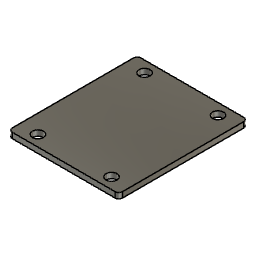
Pos34 (Autodesk Fusion 360 design; units mm, degrees)
Autodesk Fusion 360 part; units mm, degrees
sketch "Sketch1" plane through (0, 0, 0) normal (0, 0, 1) x (1, 0, 0)
  line L0 (28, -35) -> (-28, -35)
  line L1 (-30, -33) -> (-30, 33)
  line L2 (-28, 35) -> (28, 35)
  line L3 (30, 33) -> (30, -33)
  line L4 (30, -35) -> (-30, 35) construction
  line L5 (-30, -35) -> (30, 35) construction
  arc A0 (-28, 35) -> (-30, 33) centre (-28, 33) ccw
  arc A1 (30, 33) -> (28, 35) centre (28, 33) ccw
  arc A2 (28, -35) -> (30, -33) centre (28, -33) ccw
  arc A3 (-30, -33) -> (-28, -35) centre (-28, -33) ccw
  circle A4 centre (-20, -29) radius 3
  line L6 (0, 0) -> (0, -32) construction
  line L7 (0, 0) -> (-27.3192, 0) construction
  circle A5 centre (20, -29) radius 3
  circle A6 centre (-20, 29) radius 3
  circle A7 centre (20, 29) radius 3
  dimension "d1" = 60
  dimension "d2" = 70
  dimension "d3" = 2
  dimension "d4" = 6
  dimension "d5" = 10
  dimension "d6" = 6
  constraint horizontal L0
  constraint perpendicular L0 L1
  constraint parallel L0 L2
  constraint parallel L1 L3
  constraint coincident L4 L6.start
  constraint coincident L5 L6.start
  constraint coincident L6.start L7.start
  constraint coincident L4.end L2
  constraint coincident L4.end L1
  constraint tangent L2 A0
  constraint tangent L1 A0
  constraint coincident L5.end L3
  constraint coincident L5.end L2
  constraint tangent L3 A1
  constraint tangent L2 A1
  constraint equal A0 A1
  constraint coincident L4.start L3
  constraint coincident L4.start L0
  constraint tangent L3 A2
  constraint tangent L0 A2
  constraint equal A0 A2
  constraint coincident L5.start L0
  constraint coincident L5.start L1
  constraint tangent L0 A3
  constraint tangent L1 A3
  constraint equal A0 A3
  constraint vertical L6
  constraint perpendicular L6 L7
  constraint symmetric A4 L6 A5
  constraint symmetric A4 L7 A6
  constraint symmetric L7 A5 A7
  measures "d1" distance of L4.end L5.end
  measures "d2" distance of L4.start L5.end
  measures "d3" radius of A0
  measures "d4" diameter of A4
  measures "d5" distance of L1 A4.centre
  measures "d6" distance of L0 A4.centre
extrude "Extrude1" add sketch "Sketch1" along normal blind 3
